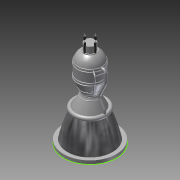
# Autodesk Inventor part: Merlin Engine
Saved by Autodesk Inventor 2015 (Build 190159000, 159)
## iProperties
Created: 2015-07-28
Part Number: Merlin Engine
Material: Generic
Document SubType Name: Modeling
Designer: Kevin
Density: 1 g/cm^3
Appearance: Steel
Author: Kevin
Autodesk Inventor part; units mm, degrees
sketch "Main" plane through (0, 0, 0) normal (0, 0, 1) x (1, 0, 0)
  line L0 (13.3848, -18.971) -> (-5.8053, -19.0152)
  arc A0 (13.3848, -18.971) -> (6.8382, -1.2269) centre (-36.7152, -27.3755) ccw
  line L1 (8.8697, 5.1439) -> (8.8697, 9.9649)
  line L2 (6.7584, -0.0759) -> (8.7683, 4.6466)
  arc A1 (6.7584, -0.0759) -> (6.8382, -1.2269) centre (7.927, -0.5732) ccw
  arc A2 (8.7683, 4.6466) -> (8.8697, 5.1439) centre (7.5997, 5.1439) ccw
  line L3 (3.7897, 14.9182) -> (3.7897, -18.9931)
  line L4 (-5.8053, -19.0152) -> (-7.068, -19.0152)
  line L5 (-7.068, -19.0152) -> (-7.068, -17.6356)
  line L6 (-7.068, -17.6356) -> (-5.5544, -17.6356)
  line L7 (3.5424, -1.6191) -> (3.5424, 13.7206)
  line L8 (3.5424, 13.7206) -> (3.7897, 13.7206)
  line L9 (2.9545, -2.28) -> (2.9545, -1.9496)
  line L10 (2.9545, -1.9496) -> (2.7115, -1.6191)
  line L11 (2.7115, -1.6191) -> (3.5424, -1.6191)
  arc A3 (-1.6133, -5.6246) -> (-2.2374, -6.9937) centre (-2.1932, -6.1871) ccw
  arc A4 (-2.2374, -6.9937) -> (-5.5629, -17.6356) centre (44.2946, -27.3755) ccw
  arc A5 (0.9224, -0.5858) -> (0.912, -0.7358) centre (0.9194, -0.661) ccw
  arc A6 (0.7413, -1.2269) -> (0.912, -0.7358) centre (-0.3476, -0.5732) ccw
  arc A7 (0.9224, -0.5858) -> (0.8512, -0.154) centre (-0.3476, -0.5732) ccw
  arc A8 (0.5141, -1.6091) -> (0.385, -1.8297) centre (0.4496, -1.7194) ccw
  arc A9 (0.7413, -1.2269) -> (0.5141, -1.6091) centre (44.2946, -27.3755) ccw
  arc A10 (0.385, -1.8297) -> (-1.6133, -5.6246) centre (44.2946, -27.3755) ccw
  arc A11 (0.7882, 0.0012) -> (0.8512, -0.154) centre (0.821, -0.0759) ccw
  arc A12 (0.1816, 1.4265) -> (0.3228, 1.0947) centre (0.2522, 1.2606) ccw
  line L12 (-1.1889, 4.6466) -> (0.1816, 1.4265)
  line L13 (0.3228, 1.0947) -> (0.7882, 0.0012)
  arc A13 (-1.2882, 5.0704) -> (-1.2157, 4.715) centre (-1.2903, 4.8849) ccw
  arc A14 (-1.2903, 5.1439) -> (-1.2882, 5.0704) centre (-0.0203, 5.1439) ccw
  arc A15 (-1.2157, 4.715) -> (-1.1889, 4.6466) centre (-0.0203, 5.1439) ccw
  arc A16 (-1.2903, 6.0236) -> (-1.2903, 5.6587) centre (-1.2903, 5.8411) ccw
  line L14 (-1.2903, 5.1439) -> (-1.2903, 5.6587)
  line L15 (-1.2903, 6.0236) -> (-1.2903, 6.5877)
  line L16 (-1.2903, 6.9525) -> (-1.2903, 9.6001)
  arc A17 (-1.2871, 9.9649) -> (-1.2903, 9.6001) centre (-1.2904, 9.7825) ccw
  arc A18 (-1.1702, 10.9289) -> (-1.2301, 10.6075) centre (-1.2028, 10.7687) ccw
  arc A19 (8.8697, 9.9649) -> (-1.1702, 10.9289) centre (3.7913, 9.8382) ccw
  arc A20 (-1.2301, 10.6075) -> (-1.2871, 9.9649) centre (3.7913, 9.8382) ccw
  line L17 (2.3323, -1.6191) -> (2.3323, -1.7193)
  line L18 (2.3323, -1.7193) -> (2.1504, -1.7193)
  line L19 (2.1504, -1.7193) -> (2.1504, -1.6191)
  line L20 (2.1504, -1.519) -> (2.3323, -1.7193) construction
  line L21 (2.3323, -1.519) -> (2.1504, -1.7193) construction
  line L22 (2.0484, -1.6191) -> (2.0484, -1.7193)
  line L23 (2.0484, -1.7193) -> (1.8666, -1.7193)
  line L24 (1.8666, -1.7193) -> (1.8666, -1.6191)
  line L25 (1.8666, -1.519) -> (2.0484, -1.7193) construction
  line L26 (2.0484, -1.519) -> (1.9575, -1.6191) construction
  line L27 (1.7694, -1.6191) -> (1.7694, -1.7193)
  line L28 (1.7694, -1.7193) -> (1.5876, -1.7193)
  line L29 (1.5876, -1.7193) -> (1.5876, -1.6191)
  line L30 (1.5876, -1.519) -> (1.7694, -1.7193) construction
  line L31 (1.7694, -1.519) -> (1.5876, -1.7193) construction
  line L32 (2.3323, -1.6191) -> (2.4685, -1.6191)
  line L33 (2.0484, -1.6191) -> (2.1504, -1.6191)
  line L34 (1.3946, -1.6191) -> (1.5876, -1.6191)
  line L35 (1.7694, -1.6191) -> (1.8666, -1.6191)
  line L36 (2.8651, -2.1585) -> (2.7973, -2.1585)
  line L37 (2.7973, -2.1585) -> (2.807, -2.0794)
  line L38 (2.7699, -2.029) -> (2.702, -2.029)
  line L39 (2.702, -2.029) -> (2.7117, -1.9499)
  line L40 (2.6753, -1.9003) -> (2.6074, -1.9003)
  line L41 (2.6074, -1.9003) -> (2.6171, -1.8213)
  line L42 (2.5663, -1.7521) -> (2.4984, -1.7521)
  line L43 (2.4984, -1.7521) -> (2.5081, -1.673)
  line L44 (2.4685, -1.6191) -> (2.5081, -1.673)
  line L45 (2.5663, -1.7521) -> (2.6171, -1.8213)
  line L46 (2.6753, -1.9003) -> (2.7117, -1.9499)
  line L47 (2.7699, -2.029) -> (2.807, -2.0794)
  line L48 (2.8651, -2.1585) -> (2.9545, -2.28)
  arc A21 (-1.9093, -5.9117) -> (-2.2148, -6.5819) centre (-2.1932, -6.1871) ccw
  line L49 (-2.2148, -6.5819) -> (-1.4728, -7.1482)
  line L50 (-1.9093, -5.9117) -> (-0.9589, -6.0231)
  arc A22 (1.3946, -1.6191) -> (-0.9589, -6.0231) centre (44.2946, -27.3755) ccw
  arc A23 (-1.4728, -7.1482) -> (-5.0398, -19.0135) centre (44.2946, -27.3755) ccw
  line L51 (-1.2903, 6.9525) -> (-1.2903, 6.5877)
  point P0 (0, 0)
  point P1 (1.6054, 0.1613)
  point P2 (5.974, 0.1613)
  point P3 (-1.2903, 2.7394)
  point P4 (8.8697, 2.7394)
  point P5 (-1.2903, 9.9649)
  point P6 (8.8697, 9.9649)
  point P7 (8.8697, 4.8849)
  point P8 (1.0766, -0.6764)
  point P9 (6.5028, -0.6764)
  point P10 (2.2414, -1.6191)
  dimension "d4" = 19.1901
  dimension "d11" = 5.08
  dimension "d13" = 5.08
  constraints: 104 end point, 51 point on circle, 24 centre point, 11 tangent, 10 horizontal, 9 parallel, 8 point on line, 5 vertical, 4 midpoint, 3 perpendicular, 1 coincident, 1 equal radius
  measures "d4" distance of L0.start L0.end
  measures "d11" distance of point (8.87, 4.885) L1.end
  measures "d13" distance of A17.start point (-1.29, 4.885)
revolve "Revolution1" add sketch "Main" angle 360 about axis through (3.7897, 14.9182, 0) along (0, -1, 0) contours L0 L4 L5 L6 A4 A3 A10 A8 A9 A6 A5 A7 A11 L13 A12 L12 A15 A13 A14 L14 A16 L15 L51 L16 A17 A20 A18 A19 L3 L8 L7 L11 L10 L9 L48 L36 L37 L47 L38 L39 L46 L40 L41 L45 L42 L43 L44 L32 L17 L18 L19 L33 L22 L23 L24 L35 L27 L28 L29 L34 A22 L50 A21 L49 A23
sketch "Sketch3" plane through (0, 0, 0) normal (0, 0, 1) x (1, 0, 0)
  line L0 (9.7727, -6.233) -> (9.7727, -4.549)
  line L1 (9.7726, -5.3793) -> (-2.1932, -5.3793) projected
  line L2 (9.589, -3.891) -> (7.824, -0.9773)
  line L3 (7.7647, 0.2291) -> (10.2093, 5.3356)
  line L4 (10.3338, 5.8839) -> (10.3338, 8.8813)
  line L5 (9.0638, 10.1513) -> (8.1605, 10.1513)
  line L6 (9.2712, -5.702) -> (9.7727, -5.702)
  arc A0 (10.3338, 8.8813) -> (9.0638, 10.1513) centre (9.0638, 8.8813) ccw
  arc A1 (10.2093, 5.3356) -> (10.3338, 5.8839) centre (9.0638, 5.8839) ccw
  arc A2 (7.7647, 0.2291) -> (7.824, -0.9773) centre (8.9103, -0.3193) ccw
  arc A3 (9.7727, -4.549) -> (9.589, -3.891) centre (8.5027, -4.549) ccw
  point P0 (0, 0)
  dimension "d19" = 1.27
  constraints: 12 end point, 8 point on circle, 8 tangent, 4 centre point, 3 equal radius, 3 perpendicular, 1 parallel, 1 point on line
  measures "d19" radius of A0
ref_plane "Work Plane1" through (9.7726, -5.3793, 0) normal (0, 1, 0) x (-1, 0, 0)
sketch "Sketch4" plane through (9.7726, -5.3793, 0) normal (0, 1, 0) x (-1, 0, 0)
  circle A0 centre (0, 0) radius 0.508
  point P0 (9.7726, 0)
  dimension "d22" = 1.016
  constraints: 1 centre point
  measures "d22" diameter of A0
sweep "Sweep1" add profiles "Sketch4" path "Sketch3" path curves L0 A3 L2 A2 L3 A1 L4 A0 L5
ref_plane "Work Plane2" through (9.7726, 14.1787, 0) normal (0, 1, 0) x (-1, 0, 0)
sketch "Sketch5" plane through (9.7726, 14.1787, 0) normal (0, 1, 0) x (-1, 0, 0)
  circle A0 centre (5.9829, 0) radius 0.2473 projected
  circle A1 centre (5.9829, 0) radius 2.6091
  point P0 (9.7726, 0)
  constraints: 1 centre point, 1 coincident
extrude "Extrusion1" add sketch "Sketch5" along normal blind 0.254
sketch "Sketch6" plane through (3.7897, 14.4327, 0) normal (0, 1, 0) x (1, 0, 0)
  circle A0 centre (0, 0) radius 2.6091
  point P0 (-3.7897, 0)
  constraints: 1 centre point
extrude "Extrusion2" cut sketch "Sketch6" along normal blind 25.4
sketch "Sketch7" plane through (3.7897, 14.4327, 0) normal (0, 1, 0) x (1, 0, 0)
  circle A0 centre (0, 0) radius 1.1823 projected
  circle A1 centre (0, 0) radius 2.2022
  circle A2 centre (0, 0) radius 2.2022 projected
  circle A3 centre (-2.2022, 0) radius 0.3492
  circle A4 centre (0, 2.2022) radius 0.3492
  line L0 (0, 0) -> (0, 2.2022)
  line L1 (0, 0) -> (2.3904, 0)
  line L2 (0, 0) -> (0, -2.5623)
  circle A5 centre (0, -2.2022) radius 0.3492
  circle A6 centre (2.2022, 0) radius 0.3492
  point P0 (-3.7897, 0)
  dimension "d28" = 0.6985
  dimension "d29" = 0.6985
  dimension "d30" = 0.6985
  dimension "d31" = 0.6985
  dimension "d51" = 4.4043
  constraints: 6 end point, 6 point on circle, 5 centre point, 2 point on line, 1 coincident, 1 horizontal, 1 vertical
  measures "d28" diameter of A3
  measures "d29" diameter of A4
  measures "d30" diameter of A5
  measures "d31" diameter of A6
  measures "d51" diameter of A1
extrude "Extrusion3" add sketch "Sketch7" along normal blind 2.54 contours L1 L0 A0 | L1 A6 A1 A5 L2 A0 | A0 L2 L1 | A0 L0 A4 A1 A6 L1 | L0 L2 A0 | A0 L2 A5 A1 A3 A4 L0 | A6 A1 L1 | L1 A1 A6 | L0 A1 A4 | A4 A1 L0 | A5 A1 L2 | L2 A1 A5 | A3 A1 picked at (0.0675, -2.0884) picked at (-0.0675, -2.0884) picked at (-2.0837, 0)
extrude "Extrusion4" add sketch "Sketch7" along normal blind 3.81 contours A6 A1 L1 | L1 A1 A6 | L0 A1 A4 | A4 A1 L0 | A5 A1 L2 | L2 A1 A5 | A1 A6 | A4 A1 | L2 A5 A1 | A1 A5 L2 | A3 A1 | A1 A3
sketch "Sketch8" plane through (1.5876, 18.2427, 0) normal (0, 1, 0) x (1, 0, 0)
  circle A0 centre (2.2022, 0) radius 2.2022 projected
  circle A1 centre (0, 0) radius 0.127
  arc A2 (1.854, 2.1745) -> (2.5503, 2.1745) centre (2.2022, 2.2022) ccw projected
  circle A3 centre (2.2022, 2.2022) radius 0.127
  circle A4 centre (4.4043, 0) radius 0.127
  circle A5 centre (2.2022, -2.2022) radius 0.127
  point P0 (-1.5876, 0)
  dimension "d36" = 0.254
  dimension "d37" = 0.254
  dimension "d38" = 0.254
  dimension "d39" = 0.254
  dimension "d50" = 4.4043
  constraints: 4 centre point, 3 point on circle, 1 coincident
  measures "d36" diameter of A1
  measures "d37" diameter of A3
  measures "d38" diameter of A4
  measures "d39" diameter of A5
  measures "d50" diameter of A0
extrude "Extrusion5" add sketch "Sketch8" along normal blind 0.635 contours A0 A4 | A0 A4 | A5 A0 | A0 A5 | A3 A0 | A0 A3 | A1 A0 | A0 A1
sketch "Sketch9" plane through (3.7897, 16.9727, 0) normal (0, 1, 0) x (1, 0, 0)
  circle A0 centre (0, 0) radius 2.6091 projected
  line L0 (2.1418, -1.49) -> (-1.9232, 1.0728)
  circle A1 centre (0, 0) radius 2.2022 projected
  point P0 (-3.7897, 0)
  constraints: 2 end point, 4 other
ref_plane "Work Plane4" through (5.9315, 16.9727, 1.49) normal (0.5333, 0, -0.8459) x (-0.8459, 0, -0.5333)
sketch "Sketch10" plane through (5.9315, 16.9727, 1.49) normal (0.5333, 0, -0.8459) x (-0.8459, 0, -0.5333)
  line L0 (-0.6389, -15.1271) -> (-1.5768, -15.1271)
  line L1 (-2.5477, -14.4105) -> (-4.444, -8.2603)
  line L2 (-3.5351, -6.9468) -> (-1.4828, -6.8215)
  arc A0 (-3.5351, -6.9468) -> (-4.444, -8.2603) centre (-3.4731, -7.9609) ccw
  arc A1 (-2.5477, -14.4105) -> (-1.5768, -15.1271) centre (-1.5768, -14.1111) ccw
  point P0 (5.8122, -16.9727)
  point P1 (-0.7433, -15.1271)
  point P2 (-1.1079, -15.1271)
  point P3 (-2.7984, -13.5974)
  point P4 (-4.3086, -7.3828)
  dimension "d44" = 1.016
  constraints: 6 end point, 5 point on circle, 4 tangent, 2 centre point, 2 point on line, 1 equal radius, 1 horizontal, 1 midpoint
  measures "d44" radius of A0
ref_plane "Work Plane5" through (8.2988, 3.3754, 2.9825) normal (0, 1, 0) x (-1, 0, 0)
sketch "Sketch11" plane through (8.2988, 3.3754, 2.9825) normal (0, 1, 0) x (-1, 0, 0)
  circle A0 centre (0, 0) radius 0.2822
  point P0 (8.2988, -2.9825)
  constraints: 1 centre point
sweep "Sweep2" add profiles "Sketch11" path "Sketch10"
ref_plane "Work Plane6" through (9.5762, 9.59, 3.7879) normal (0, 1, 0) x (-1, 0, 0)
sketch "Sketch12" plane through (9.5762, 9.59, 3.7879) normal (0, 1, 0) x (-1, 0, 0)
  line L0 (-0.1182, 0.0277) -> (-0.9651, -3.7879)
  point P0 (9.5762, -3.7879)
  constraints: 2 end point, 1 coincident
sketch "Sketch13" plane through (5.9315, 16.9727, 1.49) normal (0.5333, 0, -0.8459) x (-0.8459, 0, -0.5333)
  circle A0 centre (-4.4148, -7.4149) radius 0.1619
  point P0 (5.8122, -16.9727)
  constraints: 1 centre point
sweep "Sweep3" add profiles "Sketch13" path "Sketch12"
sketch "Sketch14" plane through (3.7897, -19.0152, 0) normal (0, -1, 0) x (1, 0, 0)
  circle A0 centre (0, 0) radius 10.8578
  point P0 (-3.7897, 0)
  constraints: 1 centre point
body "Solid1"
